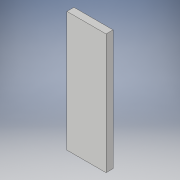
# Autodesk Inventor part: Hew Breadboard
Saved by Autodesk Inventor 2017 (Build 210142000, 142)
## iProperties
Created: 2016-10-11
Part Number: Hew Breadboard
Material: Generic
Document SubType Name: Modeling
Designer: situh
Density: 1 g/cm^3
Appearance: Default
Author: situh
Autodesk Inventor part; units mm, degrees
ref_plane "YZ Plane" through (0, 0, 0) normal (1, 0, 0) x (0, 1, 0)
ref_plane "XZ Plane" through (0, 0, 0) normal (0, 1, 0) x (-1, 0, 0)
ref_plane "XY Plane" through (0, 0, 0) normal (0, 0, 1) x (1, 0, 0)
sketch "Sketch1" plane through (0, 0, 0) normal (0, 0, 1) x (1, 0, 0)
  line L0 (-40.082, 17.3027) -> (13.6644, 17.3027)
  line L1 (13.6644, 17.3027) -> (13.6644, -147.7973)
  line L2 (13.6644, -147.7973) -> (-40.082, -147.7973)
  line L3 (-40.082, -147.7973) -> (-40.082, 17.3027)
  point P0 (0, 0)
  dimension "d0" = 165.1
  dimension "d1" = 53.7464
  constraints: 8 end point, 2 parallel, 1 horizontal, 1 perpendicular
  measures "d0" distance of L0.end L1.end
  measures "d1" distance of L0.start L0.end
extrude "Extrusion1" add sketch "Sketch1" along normal blind 9.652
body "Solid1"
